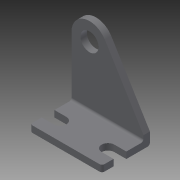
# Autodesk Inventor part: D-9969
Saved by Autodesk Inventor 2014 (Build 180170000, 170)
## iProperties
Created: 2014-01-18
Part Number: D-9969
Material: Generic
Catalog Web Link: www.cadenas.de
Description: Pivot Bracket for Original Line Cylinders - Left-
Vendor: BIMBA
Document SubType Name: Standard Catalog Part
Designer: Andrew Toennies
Manufacturer: BIMBA
Density: 1 g/cm^3
Appearance: RGB(192.00000375509219,192.00000375509219,192.00000375509219)
Category: PARTsolutions
Company: BIMBA
Title: D-9969
Author: Cadenas PARTsolutions
PSOL_IDENT_0: {$CADENAS_DATA\23d-libs\bimba\bimba\bimba_imperial\bimba_full_line\original_line_cylinders\accessori
PSOL_IDENT_1: es\pivot_bracket_left.prj},196 {VTYP=3D},{NB=D-9969},{LINA=D-9969},{NN=Pivot Bracket for Original Li
PSOL_IDENT_2: ne Cylinders - Left},{DATE=09.12.2011 06:37:01},{GEOMDATE=09.12.2011 06:36:00},{VERSION=},{LINEID=40
PSOL_IDENT_3: },{LINESUBID=-1},{WBVAR=}  {NB=D-9969},{LINA=D-9969},{KT=DUMMY},{PN=D-9969},{MAT=Zinc-Plated Carbon
PSOL_IDENT_4: Steel},{CD=0},{L=1.50000000},{L1=1.00000000},{L2=0.50000000},{L3=0.75000000},{L5=0.37500000},{L6=0.1
PSOL_IDENT_5: 3450000},{H=1.75000000},{H1=0.25000000},{H2=1.37500000},{H22=1.375},{W=1.00000000},{W1=0.26600000},{
PSOL_IDENT_6: W2=0.62500000},{R1=0.13300000},{R2=0.37500000},{R3=0.05000000},{D1=0.37750000},{C=1}
CNS_NN: Pivot Bracket for Original Line Cylinders - Left
CNS_NB: D-9969
CNS_NBSYN: $PN.
CNS_LINA: D-9969
CNS_PN: D-9969
CNS_MAT: Zinc-Plated Carbon Steel
CNS_CD: 0
CNS_L: 1.50000000
CNS_L1: 1.00000000
CNS_L2: 0.50000000
CNS_L3: 0.75000000
CNS_L5: 0.37500000
CNS_L6: 0.13450000
CNS_H: 1.75000000
CNS_H1: 0.25000000
CNS_H2: 1.37500000
CNS_H22: 1.375
CNS_W: 1.00000000
CNS_W1: 0.26600000
CNS_W2: 0.62500000
CNS_R1: 0.13300000
CNS_R2: 0.37500000
CNS_R3: 0.05000000
CNS_D1: 0.37750000
CNS_C: 1
SUPPLIER: BIMBA
ARTICLENO: D-9969
BOMINFO: D-9969
CREATOR: CADENAS GmbH
Autodesk Inventor part; units mm, degrees
ref_plane "YZ Plane" through (0, 0, 0) normal (1, 0, 0) x (0, 1, 0)
ref_plane "XZ Plane" through (0, 0, 0) normal (0, 1, 0) x (-1, 0, 0)
ref_plane "XY Plane" through (0, 0, 0) normal (0, 0, 1) x (1, 0, 0)
sketch "Sketch_1" plane through (0, 0, 0) normal (1, 0, 0) x (0, 1, 0)
  line L0 (0, 25.4) -> (0, 1.27)
  arc A0 (0, 1.27) -> (1.27, 0) centre (1.27, 1.27) ccw
  line L1 (1.27, 0) -> (44.45, 0)
  line L2 (44.45, 0) -> (44.45, 3.4163)
  line L3 (44.45, 3.4163) -> (4.6863, 3.4163)
  arc A1 (3.4163, 4.6863) -> (4.6863, 3.4163) centre (4.6863, 4.6863) ccw
  line L4 (3.4163, 4.6863) -> (3.4163, 25.4)
  line L5 (3.4163, 25.4) -> (0, 25.4)
  constraints: 12 end point, 4 point on circle, 2 centre point
extrude "Extrusion1" add sketch "Sketch_1" along normal blind 38.1
sketch "Sketch_2" plane through (0, 0, 0) normal (0, 0, 1) x (1, 0, 0)
  line L0 (-38.1, -44.45) -> (57.15, -44.45)
  line L1 (57.15, -44.45) -> (57.15, 66.675)
  line L2 (57.15, 66.675) -> (-38.1, 66.675)
  line L3 (-38.1, 66.675) -> (-38.1, -44.45)
  line L4 (0, 0) -> (38.1, 0)
  line L5 (38.1, 0) -> (38.1, 6.35)
  line L6 (38.1, 6.35) -> (17.6579, 39.8829)
  arc A0 (17.6579, 39.8829) -> (0, 34.925) centre (9.525, 34.925) ccw
  line L7 (0, 34.925) -> (0, 0)
  constraints: 16 end point, 2 point on circle, 1 centre point
extrude "Extrusion2" cut sketch "Sketch_2" along normal blind 25.4
sketch "Sketch3" plane through (38.1, 1.27, 0) normal (0, 0, -1) x (-1, 0, 0)
  point P0 (28.575, 33.655)
hole "Hole1" at (9.525, 34.925, 0) direction (0, 0, 1) diameter 9.5885 depth 3.4163
sketch "Sketch4" plane through (0, 0, 1.27) normal (0, -1, 0) x (1, 0, 0)
  point P0 (6.35, 14.605)
hole "Hole2" at (6.35, 0, 15.875) direction (0, 1, 0) diameter 6.7564 depth 3.4163
sketch "Sketch5" plane through (0, 0, 1.27) normal (0, -1, 0) x (1, 0, 0)
  point P0 (31.75, 14.605)
hole "Hole3" at (31.75, 0, 15.875) direction (0, 1, 0) diameter 6.7564 depth 3.4163
sketch "Sketch_6" plane through (0, 0, 0) normal (0, 1, 0) x (-1, 0, 0)
  line L0 (0, 12.4968) -> (0, 19.2532)
  line L1 (0, 19.2532) -> (-6.35, 19.2532)
  line L2 (-6.35, 19.2532) -> (-6.35, 12.4968)
  line L3 (-6.35, 12.4968) -> (0, 12.4968)
  constraints: 8 end point
sketch "Sketch_7" plane through (0, 0, 0) normal (0, 1, 0) x (-1, 0, 0)
  line L0 (-31.75, 12.4968) -> (-31.75, 19.2532)
  line L1 (-31.75, 19.2532) -> (-38.1, 19.2532)
  line L2 (-38.1, 19.2532) -> (-38.1, 12.4968)
  line L3 (-38.1, 12.4968) -> (-31.75, 12.4968)
  constraints: 8 end point
extrude "Extrusion3" cut sketch "Sketch_6" along normal blind 3.4163
extrude "Extrusion4" cut sketch "Sketch_7" along normal blind 3.4163
sketch "Sketch_8" plane through (0, 0, 0) normal (0, 1, 0) x (-1, 0, 0)
  line L0 (0, 38.1) -> (-38.1, 38.1)
  line L1 (-38.1, 38.1) -> (-38.1, 24.13)
  arc A0 (-36.83, 25.4) -> (-38.1, 24.13) centre (-36.83, 24.13) ccw
  line L2 (-36.83, 25.4) -> (-1.27, 25.4)
  arc A1 (0, 24.13) -> (-1.27, 25.4) centre (-1.27, 24.13) ccw
  line L3 (0, 24.13) -> (0, 38.1)
  constraints: 8 end point, 4 point on circle, 2 centre point
extrude "Extrusion5" cut sketch "Sketch_8" along normal blind 3.4163
ref_plane "a1_XY" through (0, 34.925, 0) normal (0, 0, 1) x (1, 0, 0)
ref_plane "a1_YZ" through (0, 34.925, 0) normal (1, 0, 0) x (0, 1, 0)
ref_plane "a1_ZX" through (0, 34.925, 0) normal (0, 1, 0) x (0, 0, 1)
ref_plane "a2_XY" through (9.525, 34.925, 0) normal (0, 0, 1) x (1, 0, 0)
ref_plane "a2_YZ" through (9.525, 34.925, 0) normal (1, 0, 0) x (0, 1, 0)
ref_plane "a2_ZX" through (9.525, 34.925, 0) normal (0, 1, 0) x (0, 0, 1)
ref_plane "b1_XY" through (4.7308, 34.925, 0) normal (0, 0, 1) x (1, 0, 0)
ref_plane "b1_YZ" through (4.7308, 34.925, 0) normal (1, 0, 0) x (0, 1, 0)
ref_plane "b1_ZX" through (4.7308, 34.925, 0) normal (0, 1, 0) x (0, 0, 1)
ref_plane "b2_XY" through (14.3192, 34.925, 0) normal (0, 0, 1) x (1, 0, 0)
ref_plane "b2_YZ" through (14.3192, 34.925, 0) normal (1, 0, 0) x (0, 1, 0)
ref_plane "b2_ZX" through (14.3192, 34.925, 0) normal (0, 1, 0) x (0, 0, 1)
ref_plane "d1_XY" through (0, 44.45, 0) normal (1, 0, 0) x (0, 0, -1)
ref_plane "d1_YZ" through (0, 44.45, 0) normal (0, 0, -1) x (0, 1, 0)
ref_plane "d1_ZX" through (0, 44.45, 0) normal (0, 1, 0) x (1, 0, 0)
ref_plane "d2_XY" through (0, 44.45, 3.4163) normal (1, 0, 0) x (0, 0, -1)
ref_plane "d2_YZ" through (0, 44.45, 3.4163) normal (0, 0, -1) x (0, 1, 0)
ref_plane "d2_ZX" through (0, 44.45, 3.4163) normal (0, 1, 0) x (1, 0, 0)
ref_plane "e1_XY" through (0, 0, 0) normal (0, 0, 1) x (1, 0, 0)
ref_plane "e1_YZ" through (0, 0, 0) normal (1, 0, 0) x (0, 1, 0)
ref_plane "e1_ZX" through (0, 0, 0) normal (0, 1, 0) x (0, 0, 1)
ref_plane "e2_XY" through (9.525, 44.45, 0) normal (0, 0, 1) x (1, 0, 0)
ref_plane "e2_YZ" through (9.525, 44.45, 0) normal (1, 0, 0) x (0, 1, 0)
ref_plane "e2_ZX" through (9.525, 44.45, 0) normal (0, 1, 0) x (0, 0, 1)
ref_plane "f1_XY" through (0, 0, 0) normal (0, 0, 1) x (1, 0, 0)
ref_plane "f1_YZ" through (0, 0, 0) normal (1, 0, 0) x (0, 1, 0)
ref_plane "f1_ZX" through (0, 0, 0) normal (0, 1, 0) x (0, 0, 1)
ref_plane "f2_XY" through (0, 34.925, 0) normal (0, 0, 1) x (1, 0, 0)
ref_plane "f2_YZ" through (0, 34.925, 0) normal (1, 0, 0) x (0, 1, 0)
ref_plane "f2_ZX" through (0, 34.925, 0) normal (0, 1, 0) x (0, 0, 1)
ref_plane "g1_XY" through (0, 0, 12.4968) normal (0, 1, 0) x (1, 0, 0)
ref_plane "g1_YZ" through (0, 0, 12.4968) normal (1, 0, 0) x (0, 0, -1)
ref_plane "g1_ZX" through (0, 0, 12.4968) normal (0, 0, -1) x (0, 1, 0)
ref_plane "g2_XY" through (0, 0, 19.2532) normal (0, 1, 0) x (1, 0, 0)
ref_plane "g2_YZ" through (0, 0, 19.2532) normal (1, 0, 0) x (0, 0, -1)
ref_plane "g2_ZX" through (0, 0, 19.2532) normal (0, 0, -1) x (0, 1, 0)
ref_plane "h1_XY" through (6.35, 0, 25.4) normal (0, 0, 1) x (1, 0, 0)
ref_plane "h1_YZ" through (6.35, 0, 25.4) normal (1, 0, 0) x (0, 1, 0)
ref_plane "h1_ZX" through (6.35, 0, 25.4) normal (0, 1, 0) x (0, 0, 1)
ref_plane "h2_XY" through (31.75, 0, 25.4) normal (0, 0, 1) x (1, 0, 0)
ref_plane "h2_YZ" through (31.75, 0, 25.4) normal (1, 0, 0) x (0, 1, 0)
ref_plane "h2_ZX" through (31.75, 0, 25.4) normal (0, 1, 0) x (0, 0, 1)
ref_plane "i_XY" through (38.1, 0, 25.4) normal (0, 0, 1) x (1, 0, 0)
ref_plane "i_YZ" through (38.1, 0, 25.4) normal (1, 0, 0) x (0, 1, 0)
ref_plane "i_ZX" through (38.1, 0, 25.4) normal (0, 1, 0) x (0, 0, 1)
ref_plane "j1_XY" through (0, 0, 0) normal (0, 0, 1) x (1, 0, 0)
ref_plane "j1_YZ" through (0, 0, 0) normal (1, 0, 0) x (0, 1, 0)
ref_plane "j1_ZX" through (0, 0, 0) normal (0, 1, 0) x (0, 0, 1)
ref_plane "j2_XY" through (38.1, 0, 0) normal (0, 0, 1) x (1, 0, 0)
ref_plane "j2_YZ" through (38.1, 0, 0) normal (1, 0, 0) x (0, 1, 0)
ref_plane "j2_ZX" through (38.1, 0, 0) normal (0, 1, 0) x (0, 0, 1)
ref_plane "k11_XY" through (0, 0, 25.4) normal (1, 0, 0) x (0, 0, -1)
ref_plane "k11_YZ" through (0, 0, 25.4) normal (0, 0, -1) x (0, 1, 0)
ref_plane "k11_ZX" through (0, 0, 25.4) normal (0, 1, 0) x (1, 0, 0)
ref_plane "k12_XY" through (0, 0, 0) normal (1, 0, 0) x (0, 0, -1)
ref_plane "k12_YZ" through (0, 0, 0) normal (0, 0, -1) x (0, 1, 0)
ref_plane "k12_ZX" through (0, 0, 0) normal (0, 1, 0) x (1, 0, 0)
ref_plane "to_dummy_L_XY" through (0, 0, 0) normal (0, 0, 1) x (1, 0, 0)
ref_plane "to_dummy_L_YZ" through (0, 0, 0) normal (1, 0, 0) x (0, 1, 0)
ref_plane "to_dummy_L_ZX" through (0, 0, 0) normal (0, 1, 0) x (0, 0, 1)
ref_plane "to_pin_L_XY" through (9.525, 34.925, 0) normal (0, 0, 1) x (1, 0, 0)
ref_plane "to_pin_L_YZ" through (9.525, 34.925, 0) normal (1, 0, 0) x (0, 1, 0)
ref_plane "to_pin_L_ZX" through (9.525, 34.925, 0) normal (0, 1, 0) x (0, 0, 1)
body "Solid1"
